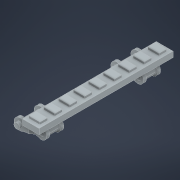
# Autodesk Inventor part: chain ink
Saved by Autodesk Inventor 2022 (Build 260153000, 153)
## iProperties
Created: 2021-12-29
Part Number: chain ink
Material: Iron, Cast
Document SubType Name: Modeling
Designer: MatusBarany
Density: 7.15 g/cm^3
Appearance: Iron Gray
Author: MatusBarany
Autodesk Inventor part; units mm, degrees
ref_plane "YZ Plane" through (0, 0, 0) normal (1, 0, 0) x (0, 1, 0)
ref_plane "XZ Plane" through (0, 0, 0) normal (0, 1, 0) x (-1, 0, 0)
sketch "Sketch2" plane through (0, 0, 0) normal (0, 0, 1) x (1, 0, 0)
  circle A0 centre (2.5, 0) radius 1.5
  circle A1 centre (-2.5, 0) radius 1.5
  arc A2 (-1.9231, 1.3846) -> (1.9231, 1.3846) centre (0, 6) ccw
  arc A3 (1.9231, -1.3846) -> (-1.9231, -1.3846) centre (0, -6) ccw
  circle A4 centre (2.5, 0) radius 0.75
  circle A5 centre (-2.5, 0) radius 0.75
  point P0 (0, 0)
  dimension "d0" = 3
  dimension "d1" = 3
  dimension "d2" = 6
  dimension "d3" = 6
  dimension "d4" = 2.5
  dimension "d5" = 2.5
  dimension "d6" = 1.5
  dimension "d7" = 1.5
  constraints: 8 point on circle, 6 centre point, 4 tangent, 2 coincident, 2 horizontal alignment
  measures "d0" diameter of A1
  measures "d1" diameter of A0
  measures "d2" distance of A2.centre point (0, 0)
  measures "d3" distance of point (0, 0) A3.centre
  measures "d4" distance of point (0, 0) A0.centre
  measures "d5" distance of A1.centre point (0, 0)
  measures "d6" diameter of A5
  measures "d7" diameter of A4
extrude "Extrusion2" add sketch "Sketch2" along normal blind 0.8
sketch "Sketch3" plane through (0, 0, 0) normal (0, 0, -1) x (-1, 0, 0)
  arc A0 (1.9231, -1.3846) -> (-1.9231, -1.3846) centre (0, -6) ccw projected
  arc A1 (1.9231, -1.3846) -> (1.9231, 1.3846) centre (2.5, 0) ccw projected
  arc A2 (-1.9231, 1.3846) -> (1.9231, 1.3846) centre (0, 6) ccw projected
  arc A3 (-1.9231, 1.3846) -> (-1.9231, -1.3846) centre (-2.5, 0) ccw projected
  circle A4 centre (-2.5, 0) radius 0.75 projected
  circle A5 centre (2.5, 0) radius 0.75 projected
  circle A6 centre (-2.5, 0) radius 1.125
  line L0 (-3.625, 2) -> (-1.375, 2)
  line L1 (-1.375, 2) -> (-1.375, 0)
  line L2 (-3.625, 0) -> (-3.625, 2)
  line L3 (0, -8.4) -> (0, 8.4) projected
  point P0 (0, 0)
  point P1 (-3.4922, 1.125)
  point P2 (-3.625, 0.9922)
  point P3 (-1.375, 1.1928)
  dimension "d12" = 2.25
  dimension "d16" = 1.5
  dimension "d20" = 2
  constraints: 6 end point, 2 parallel, 2 point on circle, 2 tangent, 1 centre point, 1 coincident, 1 perpendicular
  measures "d12" diameter of A6
  measures "d16" radius of A3
  measures "d20" distance of L0.end L1.end
extrude "Extrusion3" add sketch "Sketch3" along normal blind 1.5 contours L2 L0 L1 A2 A3 | A3 A2 L1 A6 L2 | A6
ref_plane "Work Plane1" through (-2.5, 0, -1.5) normal (0, 0, -1) x (-1, 0, 0)
sketch "Sketch4" plane through (1.375, 2, 0) normal (0, 1, 0) x (1, 0, 0)
  line L0 (-1.25, -3.5) -> (2.25, -3.5)
  line L1 (2.25, -3.5) -> (2.25, 1.5)
  line L2 (-2.75, 0) -> (-5, 0) projected
  line L3 (-2.75, 0) -> (-2.75, 3) projected
  line L4 (-2.75, 3) -> (-5, 3) projected
  line L5 (-5, 0) -> (-5, 3) projected
  line L6 (0, 0) -> (2.25, 0) projected
  line L7 (2.25, 0) -> (2.25, 1.5) projected
  line L8 (0, 0) -> (0, 1.5) projected
  line L9 (-5, 0) -> (-5, 3) projected
  line L10 (2.25, 0) -> (2.25, 3) projected
  line L11 (-1.25, 14.5) -> (2.25, 14.5)
  line L12 (2.25, 14.5) -> (2.25, 1.5)
  line L13 (-1.25, -3.5) -> (-1.25, 2.3931)
  line L14 (-1.25, 2.3931) -> (-1.25, 14.5)
  line L15 (0, 1.5) -> (2.25, 1.5) projected
  point P0 (-1.375, 0)
  point P1 (2.25, 1.5)
  dimension "d37" = 3.5
  dimension "d38" = 13
  dimension "d39" = 5
  constraints: 12 end point, 3 collinear, 2 perpendicular, 1 horizontal, 1 midpoint, 1 vertical
  measures "d37" distance of L0.start L0.end
  measures "d38" distance of L11.end L1.end
  measures "d39" distance of L0.end L1.end
extrude "Extrusion4" add sketch "Sketch4" along normal blind 1.5 contours L13 L14 L11 L12 L10 L15 L8 L6 L1 L0 | L6 L8 L15 L1
sketch "Sketch5" plane through (1.375, 3.5, 0) normal (0, 1, 0) x (1, 0, 0)
  line L0 (2.5, -0.5) -> (-0.5, -0.5)
  line L1 (-0.5, -0.5) -> (-0.5, -2.5)
  line L2 (-0.5, -2.5) -> (2.5, -2.5)
  line L3 (2.5, -2.5) -> (2.5, -0.5)
  line L4 (-1.25, -3.5) -> (2.25, -3.5) projected
  line L5 (2.25, -3.5) -> (2.25, 14.5) projected
  line L6 (2.25, 14.5) -> (-1.25, 14.5) projected
  line L7 (-1.25, 14.5) -> (-1.25, -3.5) projected
  point P0 (-1.375, 0)
  dimension "d26" = 3
  dimension "d27" = 3.5
  dimension "d28" = 2
  dimension "d30" = 1
  dimension "d84" = 0.75
  constraints: 8 end point, 2 parallel, 1 horizontal, 1 perpendicular
  measures "d26" distance of L1.end L2.end
  measures "d27" distance of L4.start L4.end
  measures "d28" distance of L0.end L1.end
  measures "d30" distance between parallel lines of L4 L2
  measures "d84" distance between parallel lines of L1 L7
extrude "Extrusion5" add sketch "Sketch5" along normal blind 0.6 contours L3 L2 L5 L0 | L5 L2 L1 L0
pattern_linear "Rectangular Pattern1" count 6 spacing 4 along (0, 0, -1) of "Extrusion5"
ref_plane "Work Plane2" through (3.625, 2, -14.5) normal (0, 0, -1) x (-1, 0, 0)
sketch "Sketch6" plane through (0, 0, 0.8) normal (0, 0, 1) x (1, 0, 0)
  arc A0 (1.9231, -1.3846) -> (-1.9231, -1.3846) centre (0, -6) ccw projected
  arc A1 (1.9231, -1.3846) -> (1.9231, 1.3846) centre (2.5, 0) ccw projected
  arc A2 (-1.9231, 1.3846) -> (1.9231, 1.3846) centre (0, 6) ccw projected
  arc A3 (-1.9231, 1.3846) -> (-1.9231, -1.3846) centre (-2.5, 0) ccw projected
  circle A4 centre (2.5, 0) radius 0.75 projected
  circle A5 centre (-2.5, 0) radius 0.75 projected
  line L0 (0, -1) -> (0, 1)
  constraints: 2 end point, 2 point on circle, 1 vertical
extrude "Extrusion6" add sketch "Sketch6" along normal blind 0.8 contours A0 A3 A2 L0
chamfer "Chamfer1" distance 0.8 angle 45 1 edges at (0, 0, 0.8)
sketch "Sketch7" plane through (0, 0, 0) normal (0, 0, -1) x (-1, 0, 0)
  line L0 (-3.625, 0) -> (-3.625, 0.9922) projected
  arc A0 (-3.625, 0.9922) -> (-1.9231, -1.3846) centre (-2.5, 0) ccw projected
  arc A1 (1.9231, -1.3846) -> (-1.9231, -1.3846) centre (0, -6) ccw projected
  arc A2 (1.9231, -1.3846) -> (1.9231, 1.3846) centre (2.5, 0) ccw projected
  arc A3 (-1.375, 1.1928) -> (1.9231, 1.3846) centre (0, 6) ccw projected
  line L1 (-1.375, 1.1928) -> (-1.375, 0) projected
  arc A4 (-3.625, 0) -> (-1.375, 0) centre (-2.5, 0) ccw projected
  circle A5 centre (2.5, 0) radius 0.75 projected
  arc A6 (-1.375, 1.1928) -> (1.9231, 1.3846) centre (0, 6) ccw projected
  line L2 (0, -1) -> (0, 1) projected
  line L3 (0, 1) -> (0, -1)
  point P0 (0, 0)
  point P1 (0, 1)
  constraints: 2 end point, 1 point on circle, 1 vertical
extrude "Extrusion7" cut sketch "Sketch7" against normal blind 0.8 contours L2 A3 A2 A1
mirror "Mirror4" about plane through (2.5, 1.4961, -1.5) normal (0, 0, -1) of "Extrusion6", "Extrusion2", "Chamfer1", "Extrusion3"
sketch "Sketch8" plane through (0, -6, -3) normal (0, 0, 1) x (1, 0, 0)
  line L0 (0, 5) -> (0, 7) projected
  line L1 (3.625, 6) -> (3.625, 6.9922) projected
  arc A0 (1.375, 6) -> (3.625, 6) centre (2.5, 6) ccw projected
  line L2 (1.375, 7.1928) -> (1.375, 6) projected
  arc A1 (-1.9231, 7.3846) -> (1.375, 7.1928) centre (0, 12) ccw projected
  arc A2 (-1.9231, 7.3846) -> (-1.9231, 4.6154) centre (-2.5, 6) ccw projected
  arc A3 (1.9231, 4.6154) -> (-1.9231, 4.6154) centre (0, 0) ccw projected
  arc A4 (1.9231, 4.6154) -> (3.625, 6.9922) centre (2.5, 6) ccw projected
  circle A5 centre (-2.5, 6) radius 0.75 projected
  point P0 (0, 6)
extrude "Extrusion8" cut sketch "Sketch8" against normal blind 0.8 contours A3 A2 A1 L0
chamfer "Chamfer3" distance 0.8 angle 45 2 edges at (0, 0, -3) (0, 0, 0)
mirror "Mirror5" about plane through (3.625, 2, -14.5) normal (0, 0, -1) of "Extrusion4", "Extrusion6", "Extrusion2", "Chamfer1", "Extrusion3", "Mirror4", "Extrusion5", "Rectangular Pattern1"
ref_plane "Work Plane3" through (3.625, 2, -14.5) normal (0, 0, -1) x (-1, 0, 0)
ref_plane "Work Plane4" through (1.375, 2, 0) normal (0, -1, 0) x (1, 0, 0)
ref_plane "Work Plane5" through (0, 0, -1.5) normal (0, 0, 1) x (1, 0, 0)
ref_plane "Work Plane6" through (1.375, 0, 0) normal (0, -1, 0) x (1, 0, 0)
sketch "Sketch9" plane through (0, 0, -1.5) normal (0, 0, 1) x (1, 0, 0)
  circle A0 centre (-2.5, 0) radius 0.75 projected
  circle A1 centre (2.5, 0) radius 0.75 projected
  line L0 (2.5, 0) -> (-2.5, 0)
  circle A2 centre (0, 0) radius 0.5
  dimension "d59" = 1
  constraints: 2 end point, 1 centre point, 1 coincident, 1 horizontal
  measures "d59" diameter of A2
sketch "Sketch10" plane through (-2.5, 0, -4.6) normal (0, 0, -1) x (-1, 0, 0)
  arc A0 (-0.5769, -1.3846) -> (-2.5, -1) centre (-2.5, -6) ccw projected
  arc A1 (-0.5769, -1.3846) -> (-0.5769, 1.3846) centre (0, 0) ccw projected
  arc A2 (-2.5, 1) -> (-0.5769, 1.3846) centre (-2.5, 6) ccw projected
  circle A3 centre (0, 0) radius 0.75 projected
  line L0 (-2.5, -1) -> (-2.5, 1) projected
  point P0 (-2.5, 0)
extrude "Extrusion9" add sketch "Sketch10" along normal blind 0.8 and the other way blind 7 contours A3
sketch "Sketch12" plane through (0, -6, -29) normal (0, 0, 1) x (1, 0, 0)
  line L0 (3.625, 6) -> (3.625, 6.9922) projected
  arc A0 (1.375, 6) -> (3.625, 6) centre (2.5, 6) ccw projected
  line L1 (1.375, 7.1928) -> (1.375, 6) projected
  arc A1 (-1.9231, 7.3846) -> (1.375, 7.1928) centre (0, 12) ccw projected
  arc A2 (-1.9231, 7.3846) -> (-1.9231, 4.6154) centre (-2.5, 6) ccw projected
  arc A3 (1.9231, 4.6154) -> (-1.9231, 4.6154) centre (0, 0) ccw projected
  arc A4 (1.9231, 4.6154) -> (3.625, 6.9922) centre (2.5, 6) ccw projected
  circle A5 centre (-2.5, 6) radius 0.75 projected
  arc A6 (-1.9231, 7.3846) -> (1.375, 7.1928) centre (0, 12) ccw projected
  line L2 (0, 7) -> (0, 5)
  point P0 (0, 6)
  constraints: 2 end point, 2 point on circle, 1 vertical
extrude "Extrusion11" cut sketch "Sketch12" along normal blind 3.8 and the other way blind 0.8 contours A3 A2 A1 L2
chamfer "Chamfer4" distance 0.8 angle 45 2 edges at (0, 0, -29) (0, 0, -26)
sketch "Sketch13" plane through (-2.5, 0, -30.6) normal (0, 0, -1) x (-1, 0, 0)
  circle A0 centre (0, 0) radius 0.75 projected
  point P0 (-2.5, 0)
extrude "Extrusion12" add sketch "Sketch13" along normal blind 0.8 and the other way blind 7
sketch "Sketch14" plane through (3.625, 2, 3.5) normal (1, 0, 0) x (0, 0, -1)
  line L0 (3.5, 0) -> (3.5, -1.0078) projected
  line L1 (3.5, -2) -> (3.5, -1.0078) projected
  line L2 (3.5, -2) -> (6.5, -2) projected
  line L3 (6.5, -2) -> (6.5, -1.0078) projected
  line L4 (6.5, 0) -> (6.5, -1.0078) projected
  line L5 (6.5, 0) -> (29.5, 0) projected
  line L6 (29.5, 0) -> (29.5, -1.0078) projected
  line L7 (29.5, -2) -> (29.5, -1.0078) projected
  line L8 (32.5, -2) -> (29.5, -2) projected
  line L9 (32.5, -2) -> (32.5, -1.0078) projected
  line L10 (32.5, 0) -> (32.5, -1.0078) projected
  line L11 (36, 0) -> (32.5, 0) projected
  line L12 (36, 0) -> (36, 1.5) projected
  line L13 (36, 1.5) -> (35, 1.5) projected
  line L14 (35, 1.5) -> (33, 1.5) projected
  line L15 (33, 1.5) -> (31, 1.5) projected
  line L16 (31, 1.5) -> (29, 1.5) projected
  line L17 (29, 1.5) -> (27, 1.5) projected
  line L18 (27, 1.5) -> (25, 1.5) projected
  line L19 (25, 1.5) -> (23, 1.5) projected
  line L20 (21, 1.5) -> (23, 1.5) projected
  line L21 (21, 1.5) -> (19, 1.5) projected
  line L22 (17, 1.5) -> (19, 1.5) projected
  line L23 (15, 1.5) -> (17, 1.5) projected
  line L24 (13, 1.5) -> (15, 1.5) projected
  line L25 (11, 1.5) -> (13, 1.5) projected
  line L26 (9, 1.5) -> (11, 1.5) projected
  line L27 (7, 1.5) -> (9, 1.5) projected
  line L28 (5, 1.5) -> (7, 1.5) projected
  line L29 (3, 1.5) -> (5, 1.5) projected
  line L30 (1, 1.5) -> (3, 1.5) projected
  line L31 (0, 1.5) -> (1, 1.5) projected
  line L32 (0, 0) -> (0, 1.5) projected
  line L33 (0, 0) -> (3.5, 0) projected
  line L34 (0, 0) -> (3.5, 0) projected
  line L35 (3.5, 0) -> (6.5, 0) projected
  line L36 (3.5, 0) -> (6.5, 0)
  line L37 (6.5, 0) -> (32.5, 0)
  constraints: 4 end point, 1 collinear, 1 horizontal
extrude "Extrusion13" add sketch "Sketch14" along normal blind 1 contours L33 L32 L31 L30 L29 L28 L27 L26 L25 L24 L23 L22 L21 L20 L19 L18 L17 L16 L15 L14 L13 L12 L11 L37 L5 L35
equation "\"d1\" = d0"
equation "\"d2\" = 2 * d0"
equation "\"d3\" = d2"
equation "\"d4\" = d5"
equation "\"d7\" = d6"
equation "\"d12\" = d16 + 0.5 * d13"
equation "\"d13\" = 1.5"
body "Solid2"
